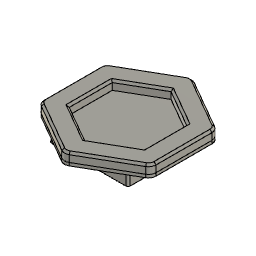
Gravitrax Duplo tower v1 (Autodesk Fusion 360 design; units mm, degrees)
Autodesk Fusion 360 part; units mm, degrees
sketch "Duplo bottom" plane through (0, 0, 0) normal (0, 0, 1) x (1, 0, 0)
  line L0 (15.85, 15.85) -> (-15.85, 15.85)
  line L1 (-15.85, 15.85) -> (-15.85, -15.85)
  line L2 (-15.85, -15.85) -> (15.85, -15.85)
  line L3 (15.85, -15.85) -> (15.85, 15.85)
  line L4 (15.85, 15.85) -> (-15.85, -15.85) construction
  line L5 (-15.85, 15.85) -> (15.85, -15.85) construction
  line L6 (14.25, -14.25) -> (14.25, 14.25)
  line L7 (14.25, 14.25) -> (-14.25, 14.25)
  line L8 (-14.25, 14.25) -> (-14.25, -14.25)
  line L9 (-14.25, -14.25) -> (14.25, -14.25)
  line L10 (12.75, -12.75) -> (-12.75, -12.75) construction
  line L11 (-12.75, -12.75) -> (-12.75, 12.75) construction
  line L12 (-12.75, 12.75) -> (12.75, 12.75) construction
  line L13 (12.75, 12.75) -> (12.75, -12.75) construction
  line L14 (12.75, -12.75) -> (-12.75, 12.75) construction
  line L15 (-12.75, -12.75) -> (12.75, 12.75) construction
  line L16 (-7.2, -12.75) -> (7.2, -12.75) construction
  line L17 (-7.2, -12.75) -> (-7.2, -14.25)
  line L18 (-7.2, -12.75) -> (-8.8, -12.75)
  line L19 (-8.8, -12.75) -> (-8.8, -14.25)
  line L20 (7.2, -12.75) -> (7.2, -14.25)
  line L21 (7.2, -12.75) -> (8.8, -12.75)
  line L22 (8.8, -12.75) -> (8.8, -14.25)
  line L23 (12.75, -8.8) -> (14.25, -8.8)
  line L24 (12.75, -7.2) -> (14.25, -7.2)
  line L25 (12.75, -7.2) -> (12.75, -8.8)
  line L26 (12.75, 7.2) -> (14.25, 7.2)
  line L27 (12.75, 8.8) -> (14.25, 8.8)
  line L28 (12.75, 7.2) -> (12.75, 8.8)
  line L29 (8.8, 12.75) -> (8.8, 14.25)
  line L30 (7.2, 12.75) -> (7.2, 14.25)
  line L31 (7.2, 12.75) -> (8.8, 12.75)
  line L32 (-7.2, 12.75) -> (-7.2, 14.25)
  line L33 (-8.8, 12.75) -> (-8.8, 14.25)
  line L34 (-7.2, 12.75) -> (-8.8, 12.75)
  line L35 (-12.75, 8.8) -> (-14.25, 8.8)
  line L36 (-12.75, 7.2) -> (-14.25, 7.2)
  line L37 (-12.75, 7.2) -> (-12.75, 8.8)
  line L38 (-12.75, -7.2) -> (-14.25, -7.2)
  line L39 (-12.75, -8.8) -> (-14.25, -8.8)
  line L40 (-12.75, -7.2) -> (-12.75, -8.8)
  circle A0 centre (0, 0) radius 6.55
  circle A1 centre (0, 0) radius 4.95
  dimension "d18" = 31.7
  dimension "d21" = 25.5
  dimension "d23" = 14.4
  dimension "d24" = 1.6
  dimension "d27" = 360
  dimension "d28" = 13.1
  constraint horizontal L0
  constraint perpendicular L0 L1
  constraint parallel L0 L2
  constraint parallel L1 L3
  constraint coincident L4 A0.centre
  constraint coincident L5 A0.centre
  constraint coincident A0.centre A1.centre
  constraint horizontal L10
  constraint perpendicular L10 L11
  constraint parallel L10 L12
  constraint parallel L11 L13
  constraint coincident L14 A0.centre
  constraint coincident L15 A0.centre
  constraint perpendicular L11 L16
  constraint midpoint L10 L16
  constraint coincident L9 L17.end
  constraint perpendicular L9 L17
  constraint coincident L10 L18.end
  constraint coincident L9 L19.end
  constraint perpendicular L9 L19
  constraint coincident L9 L20.end
  constraint perpendicular L9 L20
  constraint perpendicular L20 L21
  constraint equal L18 L21
  constraint coincident L9 L22.end
  constraint perpendicular L9 L22
  constraint equal L1 L2
  constraint equal L10 L11
  measures "d18" distance of L1.end L2.end
  measures "d21" distance of L11.end L12.end
  measures "d23" distance of L16.start L16.end
  measures "d24" distance of L16.start L18.end
  measures "d28" diameter of A0
sketch "Duplo peg" plane through (0, 0, 0) normal (0, 0, 1) x (1, 0, 0)
  line L0 (8, -8) -> (-8, -8) construction
  line L1 (-8, -8) -> (-8, 8) construction
  line L2 (-8, 8) -> (8, 8) construction
  line L3 (8, 8) -> (8, -8) construction
  line L4 (8, -8) -> (-8, 8) construction
  line L5 (-8, -8) -> (8, 8) construction
  circle A0 centre (8, 8) radius 4.75
  circle A1 centre (8, 8) radius 3.15
  circle A2 centre (-8, 8) radius 3.15
  circle A3 centre (-8, 8) radius 4.75
  circle A4 centre (-8, -8) radius 3.15
  circle A5 centre (-8, -8) radius 4.75
  circle A6 centre (8, -8) radius 3.15
  circle A7 centre (8, -8) radius 4.75
  line L6 (12.75, -12.75) -> (-12.75, -12.75) construction
  line L7 (-12.75, -12.75) -> (-12.75, 12.75) construction
  line L8 (-12.75, 12.75) -> (12.75, 12.75) construction
  line L9 (12.75, 12.75) -> (12.75, -12.75) construction
  line L10 (12.75, -12.75) -> (-12.75, 12.75) construction
  line L11 (-12.75, -12.75) -> (12.75, 12.75) construction
  dimension "d30" = 16
  dimension "d31" = 16
  dimension "d32" = 9.5
  dimension "d35" = 360
  dimension "d109" = 25.5
  dimension "d110" = 25.5
  constraint horizontal L0
  constraint perpendicular L0 L1
  constraint parallel L0 L2
  constraint parallel L1 L3
  constraint coincident L4 origin
  constraint coincident L5 origin
  constraint coincident L2.end L3.start
  constraint horizontal L6
  constraint perpendicular L6 L7
  constraint parallel L6 L8
  constraint parallel L7 L9
  constraint coincident L10 origin
  constraint coincident L11 origin
  measures "d30" distance of L1.end L2.end
  measures "d31" distance of L0.end L1.end
  measures "d32" diameter of A0
  measures "d109" distance of L7.end L8.end
  measures "d110" distance of L6.end L7.end
sketch "Gravitrax foot" plane through (0, 0, 0) normal (0, 0, 1) x (1, 0, 0)
  line L0 (14.8, 8.5448) -> (0, 17.0896)
  line L1 (0, 17.0896) -> (-14.8, 8.5448)
  line L2 (-14.8, 8.5448) -> (-14.8, -8.5448)
  line L3 (-14.8, -8.5448) -> (0, -17.0896)
  line L4 (0, -17.0896) -> (14.8, -8.5448)
  line L5 (14.8, -8.5448) -> (14.8, 8.5448)
  line L6 (22.5, 12.9904) -> (0, 25.9808)
  line L7 (0, 25.9808) -> (-22.5, 12.9904)
  line L8 (-22.5, 12.9904) -> (-22.5, -12.9904)
  line L9 (-22.5, -12.9904) -> (0, -25.9808)
  line L10 (0, -25.9808) -> (22.5, -12.9904)
  line L11 (22.5, -12.9904) -> (22.5, 12.9904)
  line L12 (13.2, 7.621) -> (0, 15.242)
  line L13 (0, 15.242) -> (-13.2, 7.621)
  line L14 (-13.2, 7.621) -> (-13.2, -7.621)
  line L15 (-13.2, -7.621) -> (0, -15.242)
  line L16 (0, -15.242) -> (13.2, -7.621)
  line L17 (13.2, -7.621) -> (13.2, 7.621)
  dimension "d36" = 14.8
  dimension "d37" = 22.5
  dimension "d38" = 13.2
  constraint vertical L11
  constraint vertical L5
  constraint vertical L17
  measures "d36" distance of origin L5
  measures "d37" distance of origin L11
  measures "d38" distance of origin L17
sketch "Gravitrax shelf" plane through (0, 0, 0) normal (0, 0, 1) x (1, 0, 0)
  line L0 (15, 8.6603) -> (0, 17.3205)
  line L1 (0, 17.3205) -> (-15, 8.6603)
  line L2 (-15, 8.6603) -> (-15, -8.6603)
  line L3 (-15, -8.6603) -> (0, -17.3205)
  line L4 (0, -17.3205) -> (15, -8.6603)
  line L5 (15, -8.6603) -> (15, 8.6603)
  line L6 (22.5, 12.9904) -> (0, 25.9808)
  line L7 (0, 25.9808) -> (-22.5, 12.9904)
  line L8 (-22.5, 12.9904) -> (-22.5, -12.9904)
  line L9 (-22.5, -12.9904) -> (0, -25.9808)
  line L10 (0, -25.9808) -> (22.5, -12.9904)
  line L11 (22.5, -12.9904) -> (22.5, 12.9904)
  line L12 (0, 0) -> (60, 0) construction
  line L13 (75, 8.6603) -> (60, 17.3205)
  line L14 (60, 17.3205) -> (45, 8.6603)
  line L15 (45, 8.6603) -> (45, -8.6603)
  line L16 (45, -8.6603) -> (60, -17.3205)
  line L17 (60, -17.3205) -> (75, -8.6603)
  line L18 (75, -8.6603) -> (75, 8.6603)
  line L19 (82.5, 12.9904) -> (60, 25.9808)
  line L20 (60, 25.9808) -> (37.5, 12.9904)
  line L21 (37.5, 12.9904) -> (37.5, -12.9904)
  line L22 (37.5, -12.9904) -> (60, -25.9808)
  line L23 (60, -25.9808) -> (82.5, -12.9904)
  line L24 (82.5, -12.9904) -> (82.5, 12.9904)
  line L25 (22.5, -12.9904) -> (37.5, -12.9904)
  line L26 (22.5, 12.9904) -> (37.5, 12.9904)
  line L27 (36.9282, 0) -> (33.4641, 6)
  line L28 (33.4641, 6) -> (26.5359, 6)
  line L29 (26.5359, 6) -> (23.0718, 0)
  line L30 (23.0718, 0) -> (26.5359, -6)
  line L31 (26.5359, -6) -> (33.4641, -6)
  line L32 (33.4641, -6) -> (36.9282, 0)
  line L33 (52.5, 38.9711) -> (52.5, 64.9519)
  line L34 (30, 25.9808) -> (52.5, 38.9711)
  line L35 (30, 34.641) -> (45, 43.3013)
  line L36 (45, 43.3013) -> (45, 60.6218)
  line L37 (45, 60.6218) -> (30, 69.282)
  line L38 (52.5, 64.9519) -> (30, 77.9423)
  line L39 (30, 77.9423) -> (7.5, 64.9519)
  line L40 (30, 69.282) -> (15, 60.6218)
  line L41 (15, 60.6218) -> (15, 43.3013)
  line L42 (15, 43.3013) -> (30, 34.641)
  line L43 (7.5, 64.9519) -> (7.5, 38.9711)
  line L44 (7.5, 38.9711) -> (30, 25.9808)
  line L45 (0, 25.9808) -> (7.5, 38.9711)
  line L46 (22.5, 12.9904) -> (30, 25.9808)
  line L47 (21.9282, 25.9808) -> (18.4641, 31.9808)
  line L48 (18.4641, 19.9808) -> (21.9282, 25.9808)
  line L49 (11.5359, 19.9808) -> (18.4641, 19.9808)
  line L50 (8.0718, 25.9808) -> (11.5359, 19.9808)
  line L51 (11.5359, 31.9808) -> (8.0718, 25.9808)
  line L52 (18.4641, 31.9808) -> (11.5359, 31.9808)
  line L53 (-7.5, 64.9519) -> (-30, 77.9423)
  line L54 (-7.5, 38.9711) -> (-7.5, 64.9519)
  line L55 (-15, 43.3013) -> (-15, 60.6218)
  line L56 (-15, 60.6218) -> (-30, 69.282)
  line L57 (-30, 69.282) -> (-45, 60.6218)
  line L58 (-30, 77.9423) -> (-52.5, 64.9519)
  line L59 (-52.5, 64.9519) -> (-52.5, 38.9711)
  line L60 (-45, 60.6218) -> (-45, 43.3013)
  line L61 (-45, 43.3013) -> (-30, 34.641)
  line L62 (-30, 34.641) -> (-15, 43.3013)
  line L63 (-52.5, 38.9711) -> (-30, 25.9808)
  line L64 (-30, 25.9808) -> (-7.5, 38.9711)
  line L65 (-22.5, 12.9904) -> (-30, 25.9808)
  line L66 (0, 25.9808) -> (-7.5, 38.9711)
  line L67 (-11.5359, 31.9808) -> (-18.4641, 31.9808)
  line L68 (-8.0718, 25.9808) -> (-11.5359, 31.9808)
  line L69 (-11.5359, 19.9808) -> (-8.0718, 25.9808)
  line L70 (-18.4641, 19.9808) -> (-11.5359, 19.9808)
  line L71 (-21.9282, 25.9808) -> (-18.4641, 19.9808)
  line L72 (-18.4641, 31.9808) -> (-21.9282, 25.9808)
  line L73 (-60, 25.9808) -> (-82.5, 12.9904)
  line L74 (-37.5, 12.9904) -> (-60, 25.9808)
  line L75 (-45, 8.6603) -> (-60, 17.3205)
  line L76 (-60, 17.3205) -> (-75, 8.6603)
  line L77 (-75, 8.6603) -> (-75, -8.6603)
  line L78 (-82.5, 12.9904) -> (-82.5, -12.9904)
  line L79 (-82.5, -12.9904) -> (-60, -25.9808)
  line L80 (-75, -8.6603) -> (-60, -17.3205)
  line L81 (-60, -17.3205) -> (-45, -8.6603)
  line L82 (-45, -8.6603) -> (-45, 8.6603)
  line L83 (-60, -25.9808) -> (-37.5, -12.9904)
  line L84 (-37.5, -12.9904) -> (-37.5, 12.9904)
  line L85 (-22.5, -12.9904) -> (-37.5, -12.9904)
  line L86 (-22.5, 12.9904) -> (-37.5, 12.9904)
  line L87 (-33.4641, 6) -> (-36.9282, 0)
  line L88 (-26.5359, 6) -> (-33.4641, 6)
  line L89 (-23.0718, 0) -> (-26.5359, 6)
  line L90 (-26.5359, -6) -> (-23.0718, 0)
  line L91 (-33.4641, -6) -> (-26.5359, -6)
  line L92 (-36.9282, 0) -> (-33.4641, -6)
  line L93 (-52.5, -38.9711) -> (-52.5, -64.9519)
  line L94 (-30, -25.9808) -> (-52.5, -38.9711)
  line L95 (-30, -34.641) -> (-45, -43.3013)
  line L96 (-45, -43.3013) -> (-45, -60.6218)
  line L97 (-45, -60.6218) -> (-30, -69.282)
  line L98 (-52.5, -64.9519) -> (-30, -77.9423)
  line L99 (-30, -77.9423) -> (-7.5, -64.9519)
  line L100 (-30, -69.282) -> (-15, -60.6218)
  line L101 (-15, -60.6218) -> (-15, -43.3013)
  line L102 (-15, -43.3013) -> (-30, -34.641)
  line L103 (-7.5, -64.9519) -> (-7.5, -38.9711)
  line L104 (-7.5, -38.9711) -> (-30, -25.9808)
  line L105 (0, -25.9808) -> (-7.5, -38.9711)
  line L106 (-22.5, -12.9904) -> (-30, -25.9808)
  line L107 (-21.9282, -25.9808) -> (-18.4641, -31.9808)
  line L108 (-18.4641, -19.9808) -> (-21.9282, -25.9808)
  line L109 (-11.5359, -19.9808) -> (-18.4641, -19.9808)
  line L110 (-8.0718, -25.9808) -> (-11.5359, -19.9808)
  line L111 (-11.5359, -31.9808) -> (-8.0718, -25.9808)
  line L112 (-18.4641, -31.9808) -> (-11.5359, -31.9808)
  line L113 (7.5, -64.9519) -> (30, -77.9423)
  line L114 (7.5, -38.9711) -> (7.5, -64.9519)
  line L115 (15, -43.3013) -> (15, -60.6218)
  line L116 (15, -60.6218) -> (30, -69.282)
  line L117 (30, -69.282) -> (45, -60.6218)
  line L118 (30, -77.9423) -> (52.5, -64.9519)
  line L119 (52.5, -64.9519) -> (52.5, -38.9711)
  line L120 (45, -60.6218) -> (45, -43.3013)
  line L121 (45, -43.3013) -> (30, -34.641)
  line L122 (30, -34.641) -> (15, -43.3013)
  line L123 (52.5, -38.9711) -> (30, -25.9808)
  line L124 (30, -25.9808) -> (7.5, -38.9711)
  line L125 (22.5, -12.9904) -> (30, -25.9808)
  line L126 (0, -25.9808) -> (7.5, -38.9711)
  line L127 (11.5359, -31.9808) -> (18.4641, -31.9808)
  line L128 (8.0718, -25.9808) -> (11.5359, -31.9808)
  line L129 (11.5359, -19.9808) -> (8.0718, -25.9808)
  line L130 (18.4641, -19.9808) -> (11.5359, -19.9808)
  line L131 (21.9282, -25.9808) -> (18.4641, -19.9808)
  line L132 (18.4641, -31.9808) -> (21.9282, -25.9808)
  line L133 (52.5, -38.9711) -> (60, -25.9808)
  line L134 (30, -25.9808) -> (37.5, -12.9904)
  line L135 (52.5, -38.9711) -> (37.5, -12.9904) construction
  line L136 (30, -25.9808) -> (60, -25.9808) construction
  line L137 (51.9282, -25.9808) -> (48.4641, -19.9808)
  line L138 (48.4641, -19.9808) -> (41.5359, -19.9808)
  line L139 (41.5359, -19.9808) -> (38.0718, -25.9808)
  line L140 (38.0718, -25.9808) -> (41.5359, -31.9808)
  line L141 (41.5359, -31.9808) -> (48.4641, -31.9808)
  line L142 (48.4641, -31.9808) -> (51.9282, -25.9808)
  line L143 (37.5, 12.9904) -> (30, 25.9808)
  line L144 (60, 25.9808) -> (52.5, 38.9711)
  line L145 (51.9282, 25.9808) -> (48.4641, 31.9808)
  line L146 (38.0718, 25.9808) -> (41.5359, 19.9808)
  line L147 (41.5359, 31.9808) -> (38.0718, 25.9808)
  line L148 (48.4641, 31.9808) -> (41.5359, 31.9808)
  line L149 (48.4641, 19.9808) -> (51.9282, 25.9808)
  line L150 (41.5359, 19.9808) -> (48.4641, 19.9808)
  line L151 (7.5, 38.9711) -> (-7.5, 38.9711)
  line L152 (7.5, 64.9519) -> (-7.5, 64.9519)
  line L153 (3.4641, 57.9615) -> (-3.4641, 57.9615)
  line L154 (-3.4641, 45.9615) -> (3.4641, 45.9615)
  line L155 (-6.9282, 51.9615) -> (-3.4641, 45.9615)
  line L156 (-3.4641, 57.9615) -> (-6.9282, 51.9615)
  line L157 (6.9282, 51.9615) -> (3.4641, 57.9615)
  line L158 (3.4641, 45.9615) -> (6.9282, 51.9615)
  line L159 (-30, 25.9808) -> (-37.5, 12.9904)
  line L160 (-52.5, 38.9711) -> (-60, 25.9808)
  line L161 (-48.4641, 31.9808) -> (-51.9282, 25.9808)
  line L162 (-41.5359, 19.9808) -> (-38.0718, 25.9808)
  line L163 (-48.4641, 19.9808) -> (-41.5359, 19.9808)
  line L164 (-51.9282, 25.9808) -> (-48.4641, 19.9808)
  line L165 (-41.5359, 31.9808) -> (-48.4641, 31.9808)
  line L166 (-38.0718, 25.9808) -> (-41.5359, 31.9808)
  line L167 (-37.5, -12.9904) -> (-30, -25.9808)
  line L168 (-60, -25.9808) -> (-52.5, -38.9711)
  line L169 (-51.9282, -25.9808) -> (-48.4641, -31.9808)
  line L170 (-38.0718, -25.9808) -> (-41.5359, -19.9808)
  line L171 (-41.5359, -31.9808) -> (-38.0718, -25.9808)
  line L172 (-48.4641, -31.9808) -> (-41.5359, -31.9808)
  line L173 (-48.4641, -19.9808) -> (-51.9282, -25.9808)
  line L174 (-41.5359, -19.9808) -> (-48.4641, -19.9808)
  line L175 (-7.5, -38.9711) -> (7.5, -38.9711)
  line L176 (-7.5, -64.9519) -> (7.5, -64.9519)
  line L177 (-3.4641, -57.9615) -> (3.4641, -57.9615)
  line L178 (3.4641, -45.9615) -> (-3.4641, -45.9615)
  line L179 (6.9282, -51.9615) -> (3.4641, -45.9615)
  line L180 (3.4641, -57.9615) -> (6.9282, -51.9615)
  line L181 (-6.9282, -51.9615) -> (-3.4641, -57.9615)
  line L182 (-3.4641, -45.9615) -> (-6.9282, -51.9615)
  point P0 (60, 0)
  point P1 (60, 0)
  point P2 (30, 0)
  point P3 (45, -25.9808)
  dimension "d39" = 15
  dimension "d40" = 22.5
  dimension "d41" = 60
  dimension "d43" = 15
  dimension "d44" = 22.5
  dimension "d45" = 6
  dimension "d47" = 360
  dimension "d48" = 6
  dimension "d50" = 360
  constraint coincident L12.start origin
  constraint horizontal L12
  constraint coincident P1 P0
  constraint vertical L24
  constraint vertical L18
  constraint vertical L11
  constraint vertical L5
  constraint midpoint L12 P2
  constraint horizontal L31
  constraint midpoint L135 P3
  constraint horizontal L138
  measures "d39" distance of L12.start L5
  measures "d40" distance of L12.start L11
  measures "d41" distance of L12.start P1
  measures "d43" distance of P1 L18
  measures "d44" distance of P1 L24
  measures "d45" distance of P2 L32
  measures "d48" distance of P3 L142
extrude "Extrude1" add sketch "Gravitrax foot" against normal blind 1.2 contours L0 L1 L2 L3 L4 L5 | L6 L7 L8 L9 L10 L11 makes body 1
extrude "Extrude2" add sketch "Gravitrax foot" against normal blind 3 from surface at -1.2 contours L0 L1 L2 L3 L4 L5 bodies 1
fillet "Fillet1" radius 3 6 edges at (22.5, 12.9904, -0.6) (22.5, -12.9904, -0.6) (0, -25.9808, -0.6) (0, 25.9808, -0.6) (-22.5, 12.9904, -0.6) (-22.5, -12.9904, -0.6) on bodies 1
fillet "Fillet1" radius 0.8 6 edges at (-13.2, 0, 0) (-6.6, -11.4315, 0) (6.6, -11.4315, 0) (13.2, 0, 0) (6.6, 11.4315, 0) (-6.6, 11.4315, 0) on bodies 1
fillet "Fillet1" radius 0.8 1 faces at (-14.2667, 2.5403, -4.2) on bodies 1
fillet "Fillet1" radius 0.8 6 edges at (-14.8, -8.5448, -2.7) (-14.8, 8.5448, -2.7) (0, -17.0896, -2.7) (14.8, -8.5448, -2.7) (14.8, 8.5448, -2.7) (0, 17.0896, -2.7) on bodies 1
fillet "Fillet1" radius 1.6 6 edges at (13.2, -7.621, -2.1) (13.2, 7.621, -2.1) (0, 15.242, -2.1) (-13.2, 7.621, -2.1) (-13.2, -7.621, -2.1) (0, -15.242, -2.1) on bodies 1
extrude "Extrude3" add sketch "Gravitrax foot" along normal blind 1.2 separate body contours L0 L1 L2 L3 L4 L5 | L6 L7 L8 L9 L10 L11 | L12 L13 L14 L15 L16 L17 makes body 2
extrude "Extrude4" add sketch "Duplo peg" along normal blind 5.7 bodies 2
fillet "Fillet2" radius 3 6 edges at (22.5, -12.9904, 0.6) (0, -25.9808, 0.6) (-22.5, -12.9904, 0.6) (22.5, 12.9904, 0.6) (-22.5, 12.9904, 0.6) (0, 25.9808, 0.6) on bodies 2
fillet "Fillet2" radius 0.8 4 edges at (-12.4286, 6.2823, 5.7) (3.5714, 6.2823, 5.7) (3.5714, -9.7177, 5.7) (-12.4286, -9.7177, 5.7) on bodies 2
fillet "Fillet2" radius 0.8 4 edges at (-10.9368, 6.8609, 1.2) (5.0632, 6.8609, 1.2) (5.0632, -9.1391, 1.2) (-10.9368, -9.1391, 1.2) on bodies 2
extrude "Extrude6" add sketch "Gravitrax shelf" against normal blind 1.2 separate body contours L0 L1 L2 L3 L4 L5 | L6 L7 L8 L9 L10 L11 makes body 3
extrude "Extrude5" add sketch "Duplo bottom" against normal blind 6.1 contours L0 L1 L2 L3 | L6 L23 L24 L25 | L9 L20 L21 L22 | L6 L26 L27 L28 | L9 L17 L18 L19 | L7 L29 L30 L31 | L8 L38 L39 L40 | L7 L32 L33 L34 | L8 L35 L36 L37 | A0 bodies 3
fillet "Fillet3" radius 3 6 edges at (0, -25.9808, -0.6) (22.5, -12.9904, -0.6) (-22.5, -12.9904, -0.6) (22.5, 12.9904, -0.6) (0, 25.9808, -0.6) (-22.5, 12.9904, -0.6) on bodies 3
fillet "Fillet3" radius 0.8 1 faces at (0.1632, -11.6772, -1.2) on bodies 3
fillet "Fillet3" radius 0.8 4 edges at (0, 15.85, -1.2) (-15.85, 0, -1.2) (15.85, 0, -1.2) (0, -15.85, -1.2) on bodies 3
fillet "Fillet3" radius 0.8 1 edges at (-4.615, 1.79, -1.2) on bodies 3
fillet "Fillet3" radius 0.8 4 edges at (15.85, -15.85, -3.65) (-15.85, -15.85, -3.65) (-15.85, 15.85, -3.65) (15.85, 15.85, -3.65) on bodies 3
extrude "Extrude8" add sketch "Gravitrax shelf" along normal blind 3.5 separate body contours L6 L7 L8 L9 L10 L11 makes body 4
fillet "Fillet4" radius 3 6 edges at (-22.5, 12.9904, 1.75) (0, 25.9808, 1.75) (-22.5, -12.9904, 1.75) (0, -25.9808, 1.75) (22.5, -12.9904, 1.75) (22.5, 12.9904, 1.75) on bodies 4
chamfer "Chamfer1" distance 0.8 angle 45 1 faces at (7.5, 18.7639, 3.5) on bodies 4
extrude "Extrude13" add sketch "Gravitrax shelf" along normal blind 1.75 separate body contours L6 L7 L8 L9 L10 L11 | L11 L21 L25 L26 | L19 L20 L21 L22 L23 L24 makes body 5
extrude "Extrude14" add sketch "Gravitrax shelf" along normal blind 3.5 contours L6 L7 L8 L9 L10 L11 | L19 L20 L21 L22 L23 L24 bodies 5
fillet "Fillet10" radius 0.5333 7 edges at (48.75, -19.4856, 0) (71.25, -19.4856, 0) (30, -12.9904, 0) (82.5, 0, 0) (71.25, 19.4856, 0) (48.75, 19.4856, 0) (30, 12.9904, 0) on bodies 5
fillet "Fillet10" radius 3 8 edges at (82.5, 12.9904, 1.75) (82.5, -12.9904, 1.75) (60, -25.9808, 1.75) (0, -25.9808, 1.75) (-22.5, -12.9904, 1.75) (-22.5, 12.9904, 1.75) (0, 25.9808, 1.75) (60, 25.9808, 1.75) on bodies 5
chamfer "Chamfer7" distance 0.8 angle 45 2 faces at (20, -2.8868, 3.5) (40, -2.8868, 3.5) on bodies 5
extrude "Extrude15" add sketch "Gravitrax shelf" along normal blind 1.75 separate body contours L6 L7 L8 L9 L10 L11 | L11 L21 L25 L26 | L19 L20 L21 L22 L23 L24 | L8 L84 L85 L86 | L73 L74 L78 L79 L83 L84 makes body 6
extrude "Extrude16" add sketch "Gravitrax shelf" along normal blind 3.5 contours L6 L7 L8 L9 L10 L11 | L19 L20 L21 L22 L23 L24 | L73 L74 L78 L79 L83 L84 bodies 6
fillet "Fillet9" radius 3 10 edges at (60, 25.9808, 1.75) (82.5, 12.9904, 1.75) (82.5, -12.9904, 1.75) (60, -25.9808, 1.75) (0, -25.9808, 1.75) (-60, -25.9808, 1.75) (0, 25.9808, 1.75) (-60, 25.9808, 1.75) (-82.5, 12.9904, 1.75) (-82.5, -12.9904, 1.75) on bodies 6
fillet "Fillet9" radius 0.5333 14 edges at (-71.25, 19.4856, 0) (-48.75, 19.4856, 0) (-30, 12.9904, 0) (-30, -12.9904, 0) (-48.75, -19.4856, 0) (-71.25, -19.4856, 0) (-82.5, 0, 0) (30, -12.9904, 0) (30, 12.9904, 0) (48.75, 19.4856, 0) (71.25, 19.4856, 0) (82.5, 0, 0) (71.25, -19.4856, 0) (48.75, -19.4856, 0) on bodies 6
chamfer "Chamfer6" distance 0.8 angle 45 3 faces at (40, -2.8868, 3.5) (-20, 2.8868, 3.5) (-40, 2.8868, 3.5) on bodies 6
extrude "Extrude17" add sketch "Gravitrax shelf" along normal blind 1.75 separate body contours L6 L7 L8 L9 L10 L11 | L11 L21 L25 L26 | L7 L64 L65 L66 | L19 L20 L21 L22 L23 L24 | L53 L54 L58 L59 L63 L64 | L9 L104 L105 L106 | L93 L94 L98 L99 L103 L104 makes body 7
extrude "Extrude18" add sketch "Gravitrax shelf" along normal blind 3.5 contours L6 L7 L8 L9 L10 L11 | L19 L20 L21 L22 L23 L24 | L53 L54 L58 L59 L63 L64 | L93 L94 L98 L99 L103 L104 bodies 7
fillet "Fillet8" radius 3 12 edges at (-7.5, -64.9519, 1.75) (-30, -77.9423, 1.75) (-52.5, -64.9519, 1.75) (-52.5, -38.9711, 1.75) (-52.5, 38.9711, 1.75) (-52.5, 64.9519, 1.75) (-30, 77.9423, 1.75) (-7.5, 64.9519, 1.75) (60, 25.9808, 1.75) (82.5, 12.9904, 1.75) (82.5, -12.9904, 1.75) (60, -25.9808, 1.75) on bodies 7
fillet "Fillet8" radius 0.5333 21 edges at (-7.5, 51.9615, 0) (-18.75, 71.4471, 0) (-41.25, 71.4471, 0) (-52.5, 51.9615, 0) (-41.25, 32.476, 0) (-26.25, 19.4856, 0) (-3.75, 32.476, 0) (-26.25, -19.4856, 0) (-3.75, -32.476, 0) (-7.5, -51.9615, 0) (-18.75, -71.4471, 0) (-41.25, -32.476, 0) (-52.5, -51.9615, 0) (-41.25, -71.4471, 0) (30, -12.9904, 0) (30, 12.9904, 0) (48.75, -19.4856, 0) (71.25, -19.4856, 0) (82.5, 0, 0) (71.25, 19.4856, 0) (48.75, 19.4856, 0) on bodies 7
chamfer "Chamfer5" distance 0.8 angle 45 4 faces at (-17.5, 36.0844, 3.5) (-22.5, -33.1976, 3.5) (7.5, 18.7639, 3.5) (40, -2.8868, 3.5) on bodies 7
hidden bodies 1 2 5 6 7
equation "Duplo_brick_width = 31,7 mm" comment "External dimensions of a 2x2 Duplo brick."
equation "Duplo_center_diameter = 13,2 mm" comment "Diameter of the circle inside a 2x2 Duplo block."
equation "Duplo_inset = Duplo_pin_height + 0,4 mm" comment "The height of the space for the Duplo pin."
equation "Duplo_pin_diameter = 9,5 mm"
equation "Duplo_pin_distance = 16 mm"
equation "Duplo_pin_height = 4,5 mm"
equation "Duplo_margin = 0,1 mm"
equation "Wall_thickness = 1,6 mm"
equation "Gravitrax_block_distance = 60 mm" comment "Distance between Gravitrax bulding elements."
equation "Gravitrax_spacer_height = Gravitrax_foot_height + 0,5 mm"
equation "Gravitrax_plate_hole = 30 mm"
equation "Gravitrax_margin = 0,2 mm"
equation "Gravitrax_foot_height = 3 mm"
equation "Gravitrax_outside_dimensions = 45 mm"
equation "Separator_wall_thickness = 1,2 mm" comment "The thickness of the separation between the Duplo connector and the Gravitrax connector."
equation "d18 = Duplo_brick_width"
equation "d20 = -Wall_thickness"
equation "d21 = Duplo_pin_distance + Duplo_pin_diameter"
equation "d23 = Duplo_pin_distance - Wall_thickness"
equation "d28 = Duplo_center_diameter - Duplo_margin"
equation "d29 = -Wall_thickness"
equation "d30 = Duplo_pin_distance"
equation "d31 = Duplo_pin_distance"
equation "d32 = Duplo_pin_diameter"
equation "d33 = -Wall_thickness"
equation "d36 = ( Gravitrax_plate_hole ) / 2 - Gravitrax_margin"
equation "d37 = Gravitrax_outside_dimensions / 2"
equation "d38 = ( Gravitrax_plate_hole ) / 2 - Gravitrax_margin - Wall_thickness"
equation "d39 = Gravitrax_plate_hole / 2"
equation "d40 = Gravitrax_outside_dimensions / 2"
equation "d41 = Gravitrax_block_distance"
equation "d43 = Gravitrax_plate_hole / 2"
equation "d44 = Gravitrax_outside_dimensions / 2"
equation "d51 = -Separator_wall_thickness"
equation "d53 = -Gravitrax_foot_height"
equation "d55 = Separator_wall_thickness"
equation "d57 = Separator_wall_thickness + Duplo_pin_height"
equation "d59 = -Separator_wall_thickness - Duplo_inset"
equation "d61 = -Separator_wall_thickness"
equation "d65 = Gravitrax_spacer_height"
equation "d68 = Corner_fillet"
equation "d70 = Wall_thickness / 2"
equation "d72 = Wall_thickness / 2"
equation "d74 = Wall_thickness / 2"
equation "d76 = Wall_thickness"
equation "d78 = Corner_fillet"
equation "d80 = Wall_thickness / 2"
equation "d82 = Wall_thickness / 2"
equation "d84 = Corner_fillet"
equation "d86 = Wall_thickness / 2"
equation "d88 = Wall_thickness / 2"
equation "d90 = Wall_thickness / 2"
equation "d92 = Corner_fillet"
equation "d93 = Wall_thickness / 2"
equation "d95 = Wall_thickness / 2"
equation "Duplo_brick_hight = 19,1 mm"
equation "d109 = Duplo_pin_distance + Duplo_pin_diameter"
equation "d110 = Duplo_pin_distance + Duplo_pin_diameter"
equation "d121 = Gravitrax_spacer_height / 2"
equation "d123 = Gravitrax_spacer_height"
equation "d125 = Gravitrax_spacer_height / 2"
equation "d127 = Gravitrax_spacer_height"
equation "d129 = Gravitrax_spacer_height / 2"
equation "d131 = Gravitrax_spacer_height"
equation "d133 = Wall_thickness / 2"
equation "d135 = Corner_fillet"
equation "d137 = Wall_thickness / 3"
equation "d139 = Corner_fillet"
equation "d141 = Wall_thickness / 3"
equation "d142 = Wall_thickness / 2"
equation "d144 = Wall_thickness / 3"
equation "d146 = Corner_fillet"
equation "d147 = Wall_thickness / 2"
equation "Corner_fillet = 3 mm"
equation "d149 = -Separator_wall_thickness"
named bodies: "Base-Gravitrax foot", "Base-Duplo peg", "Spacer-Duplo", "Spacer-towertop", "Spacer-single-shelf", "Spacer-duo-shelf", "Spacer-tri-shelf"
